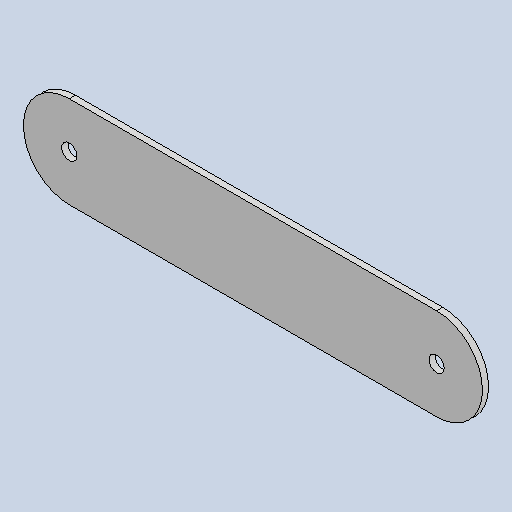
# Autodesk Inventor part: ДМФ 01 15 Барабан усилитель борта
Saved by Autodesk Inventor 2026.2 (Build 302298010, 298A)
## iProperties
Created: 2024-04-30
Part Number: ДМФ 01 15 Барабан усилитель борта
Material: Generic
Document SubType Name: Sheet Metal
Designer: pokla
Stock Number: Барабан_Сектор_Усилителя
Density: 1 g/cm^3
Flat Pattern Width: 7.5922 cm
Flat Pattern Length: 14.0866 cm
Flat Pattern Area: 106.948 cm^2
Sheet Metal Rule: Default
Sheet Metal Width: 75,922 mm
Sheet Metal Length: 140,866 mm
Sheet Metal Area: 10694,795 mm^2
Appearance: Default
Author: pokla
Autodesk Inventor part; units mm, degrees
ref_plane "YZ Plane" through (0, 0, 0) normal (1, 0, 0) x (0, 1, 0)
ref_plane "XZ Plane" through (0, 0, 0) normal (0, 1, 0) x (-1, 0, 0)
ref_plane "XY Plane" through (0, 0, 0) normal (0, 0, 1) x (1, 0, 0)
sketch "Sketch1" plane through (0, 0, 0) normal (0, 0, 1) x (1, 0, 0)
  line L0 (-60, 0) -> (60, 0) construction
  line L1 (-60, -15) -> (60, -15)
  line L2 (60, 15) -> (-60, 15)
  arc A0 (-60, 15) -> (-60, -15) centre (-60, 0) ccw
  arc A1 (60, -15) -> (60, 15) centre (60, 0) ccw
  circle A2 centre (-60, 0) radius 2.5
  circle A3 centre (60, 0) radius 2.5
  line L3 (0, 15) -> (0, -15) construction
  point P0 (0, 0)
  point P1 (0, 0)
  point P2 (0, 0)
  point P3 (0, 0)
  dimension "d37" = 120
  dimension "d38" = 15
  dimension "d39" = 120
  dimension "d40" = 5
  measures "d37" distance of L0.start L0.end
  measures "d38" radius of A1
  measures "d39" distance of A3.centre A2.centre
  measures "d40" diameter of A2
extrude "Plate1" add sketch "Sketch1" against normal blind 2
equation "\"d15\" = Thickness"
equation "\"BendRadius\" = Thickness"
equation "\"BendReliefWidth\" = Thickness"
equation "\"BendReliefDepth\" = 0.5 * Thickness"
equation "\"CornerReliefSize\" = 4 * Thickness"
equation "\"MinimumRemnant\" = 2 * Thickness"
equation "\"TransitionRadius\" = BendRadius"
equation "\"JacobiRadiusSize\" = BendRadius"
equation "\"GapSize\" = Thickness"
equation "\"Thickness\" = 2"
body "Solid1"
